Autodesk Inventor part; units mm, degrees
(part 4 of 4)
  spline S72 degree 5 poles (-3.5929, 3.9724) (-3.5942, 3.9738) (-3.5967, 3.9765) (-3.6006, 3.9805) (-3.6059, 3.9857) (-3.6128, 3.9919) (-3.6198, 3.998) (-3.627, 4.004) (-3.6342, 4.01) (-3.6414, 4.0159) (-3.6487, 4.0217) (-3.6561, 4.0275) (-3.6635, 4.0333) (-3.671, 4.039) (-3.6786, 4.0446) (-3.6863, 4.0501) (-3.694, 4.0556) (-3.7017, 4.061) (-3.7095, 4.0663) (-3.7174, 4.0716) (-3.7253, 4.0769) (-3.7333, 4.0821) (-3.7413, 4.0873) (-3.7493, 4.0925) (-3.7574, 4.0976) (-3.7656, 4.1026) (-3.7738, 4.1076) (-3.782, 4.1125) (-3.7903, 4.1174) (-3.7986, 4.1223) (-3.8069, 4.1271) (-3.8153, 4.1319) (-3.8237, 4.1367) (-3.8322, 4.1414) (-3.8407, 4.146) (-3.8493, 4.1507) (-3.8578, 4.1552) (-3.8665, 4.1598) (-3.8751, 4.1643) (-3.8838, 4.1688) (-3.8925, 4.1732) (-3.9013, 4.1776) (-3.9101, 4.182) (-3.9189, 4.1863) (-3.9278, 4.1906) (-3.9366, 4.1948) (-3.9456, 4.199) (-3.9545, 4.2032) (-3.9635, 4.2074) (-3.9725, 4.2115) (-3.9816, 4.2156) (-3.9907, 4.2196) (-3.9998, 4.2236) (-4.0089, 4.2276) (-4.0181, 4.2315) (-4.0273, 4.2354) (-4.0365, 4.2393) (-4.0458, 4.2431) (-4.0551, 4.2469) (-4.0644, 4.2507) (-4.0737, 4.2544) (-4.0831, 4.2581) (-4.0925, 4.2618) (-4.1019, 4.2654) (-4.1114, 4.269) (-4.1208, 4.2726) (-4.1304, 4.2761) (-4.1399, 4.2796) (-4.1533, 4.2845) (-4.1648, 4.2886) (-4.1744, 4.2919) (-4.1822, 4.2946) (-4.188, 4.2966) knots 0 0 0 0 0 0 0.014286 0.028571 0.042857 0.057143 0.071429 0.085714 0.1 0.114286 0.128571 0.142857 0.157143 0.171429 0.185714 0.2 0.214286 0.228571 0.242857 0.257143 0.271429 0.285714 0.3 0.314286 0.328571 0.342857 0.357143 0.371429 0.385714 0.4 0.414286 0.428571 0.442857 0.457143 0.471429 0.485714 0.5 0.514286 0.528571 0.542857 0.557143 0.571429 0.585714 0.6 0.614286 0.628571 0.642857 0.657143 0.671429 0.685714 0.7 0.714286 0.728571 0.742857 0.757143 0.771429 0.785714 0.8 0.814286 0.828571 0.842857 0.857143 0.871429 0.885714 0.9 0.914286 0.928571 0.942857 0.957143 1 1 1 1 1 1
  arc A73 (-4.188, 4.2966) -> (-4.3439, 4.1389) centre (0, 0) ccw
  spline S73 degree 5 poles (-4.013, 3.5476) (-4.0144, 3.5488) (-4.0171, 3.5513) (-4.0212, 3.5552) (-4.0264, 3.5604) (-4.0327, 3.5672) (-4.0389, 3.5742) (-4.045, 3.5813) (-4.051, 3.5884) (-4.057, 3.5956) (-4.0629, 3.6028) (-4.0688, 3.6101) (-4.0746, 3.6175) (-4.0804, 3.6249) (-4.0861, 3.6324) (-4.0917, 3.64) (-4.0972, 3.6477) (-4.1027, 3.6554) (-4.1082, 3.6631) (-4.1136, 3.6709) (-4.119, 3.6788) (-4.1243, 3.6867) (-4.1296, 3.6946) (-4.1348, 3.7026) (-4.14, 3.7106) (-4.1451, 3.7187) (-4.1502, 3.7269) (-4.1552, 3.735) (-4.1602, 3.7432) (-4.1652, 3.7515) (-4.1701, 3.7598) (-4.175, 3.7681) (-4.1798, 3.7765) (-4.1846, 3.7849) (-4.1894, 3.7934) (-4.1941, 3.8019) (-4.1988, 3.8104) (-4.2034, 3.819) (-4.208, 3.8276) (-4.2126, 3.8362) (-4.2172, 3.8449) (-4.2216, 3.8536) (-4.2261, 3.8623) (-4.2305, 3.8711) (-4.2349, 3.8799) (-4.2393, 3.8887) (-4.2436, 3.8976) (-4.2479, 3.9065) (-4.2521, 3.9155) (-4.2563, 3.9244) (-4.2605, 3.9334) (-4.2646, 3.9425) (-4.2688, 3.9515) (-4.2728, 3.9606) (-4.2769, 3.9698) (-4.2809, 3.9789) (-4.2848, 3.9881) (-4.2888, 3.9973) (-4.2927, 4.0066) (-4.2966, 4.0158) (-4.3004, 4.0251) (-4.3042, 4.0345) (-4.308, 4.0438) (-4.3117, 4.0532) (-4.3154, 4.0626) (-4.3191, 4.0721) (-4.3227, 4.0815) (-4.3264, 4.091) (-4.3314, 4.1043) (-4.3356, 4.1158) (-4.3391, 4.1254) (-4.3418, 4.1331) (-4.3439, 4.1389) knots 0 0 0 0 0 0 0.014286 0.028571 0.042857 0.057143 0.071429 0.085714 0.1 0.114286 0.128571 0.142857 0.157143 0.171429 0.185714 0.2 0.214286 0.228571 0.242857 0.257143 0.271429 0.285714 0.3 0.314286 0.328571 0.342857 0.357143 0.371429 0.385714 0.4 0.414286 0.428571 0.442857 0.457143 0.471429 0.485714 0.5 0.514286 0.528571 0.542857 0.557143 0.571429 0.585714 0.6 0.614286 0.628571 0.642857 0.657143 0.671429 0.685714 0.7 0.714286 0.728571 0.742857 0.757143 0.771429 0.785714 0.8 0.814286 0.828571 0.842857 0.857143 0.871429 0.885714 0.9 0.914286 0.928571 0.942857 0.957143 1 1 1 1 1 1
  line L73 (-3.9631, 3.5028) -> (-4.013, 3.5476)
  arc A74 (-3.9631, 3.5028) -> (-4.1449, 3.2856) centre (0, 0) ccw
  line L74 (-4.1449, 3.2856) -> (-4.1978, 3.3269)
  spline S74 degree 5 poles (-4.1978, 3.3269) (-4.1992, 3.328) (-4.2022, 3.3303) (-4.2067, 3.3336) (-4.2128, 3.3378) (-4.2206, 3.3429) (-4.2285, 3.3477) (-4.2365, 3.3524) (-4.2446, 3.3571) (-4.2528, 3.3617) (-4.2609, 3.3663) (-4.2691, 3.3708) (-4.2774, 3.3753) (-4.2858, 3.3797) (-4.2941, 3.3839) (-4.3026, 3.3881) (-4.3111, 3.3922) (-4.3197, 3.3963) (-4.3283, 3.4003) (-4.3369, 3.4042) (-4.3455, 3.4081) (-4.3543, 3.412) (-4.363, 3.4158) (-4.3718, 3.4195) (-4.3806, 3.4232) (-4.3895, 3.4268) (-4.3984, 3.4304) (-4.4073, 3.4339) (-4.4163, 3.4374) (-4.4253, 3.4409) (-4.4343, 3.4442) (-4.4434, 3.4476) (-4.4525, 3.4509) (-4.4616, 3.4541) (-4.4707, 3.4573) (-4.4799, 3.4605) (-4.4892, 3.4636) (-4.4984, 3.4667) (-4.5077, 3.4697) (-4.517, 3.4727) (-4.5263, 3.4756) (-4.5357, 3.4785) (-4.5451, 3.4814) (-4.5545, 3.4842) (-4.5639, 3.4869) (-4.5734, 3.4897) (-4.5829, 3.4924) (-4.5924, 3.495) (-4.602, 3.4976) (-4.6115, 3.5002) (-4.6211, 3.5027) (-4.6308, 3.5052) (-4.6404, 3.5077) (-4.6501, 3.5101) (-4.6598, 3.5124) (-4.6695, 3.5148) (-4.6792, 3.5171) (-4.689, 3.5193) (-4.6988, 3.5215) (-4.7086, 3.5237) (-4.7184, 3.5259) (-4.7283, 3.528) (-4.7381, 3.53) (-4.748, 3.5321) (-4.7579, 3.5341) (-4.7679, 3.536) (-4.7778, 3.5379) (-4.7878, 3.5398) (-4.8018, 3.5424) (-4.8139, 3.5446) (-4.8239, 3.5463) (-4.832, 3.5477) (-4.8381, 3.5487) knots 0 0 0 0 0 0 0.014286 0.028571 0.042857 0.057143 0.071429 0.085714 0.1 0.114286 0.128571 0.142857 0.157143 0.171429 0.185714 0.2 0.214286 0.228571 0.242857 0.257143 0.271429 0.285714 0.3 0.314286 0.328571 0.342857 0.357143 0.371429 0.385714 0.4 0.414286 0.428571 0.442857 0.457143 0.471429 0.485714 0.5 0.514286 0.528571 0.542857 0.557143 0.571429 0.585714 0.6 0.614286 0.628571 0.642857 0.657143 0.671429 0.685714 0.7 0.714286 0.728571 0.742857 0.757143 0.771429 0.785714 0.8 0.814286 0.828571 0.842857 0.857143 0.871429 0.885714 0.9 0.914286 0.928571 0.942857 0.957143 1 1 1 1 1 1
  arc A75 (-4.8381, 3.5487) -> (-4.9659, 3.3675) centre (0, 0) ccw
  spline S75 degree 5 poles (-4.5422, 2.8387) (-4.5437, 2.8397) (-4.5469, 2.8417) (-4.5515, 2.8448) (-4.5575, 2.8492) (-4.5649, 2.8548) (-4.5721, 2.8607) (-4.5793, 2.8666) (-4.5864, 2.8727) (-4.5935, 2.8788) (-4.6005, 2.8849) (-4.6075, 2.8912) (-4.6145, 2.8975) (-4.6214, 2.9039) (-4.6282, 2.9103) (-4.635, 2.9169) (-4.6418, 2.9235) (-4.6484, 2.9302) (-4.6551, 2.937) (-4.6617, 2.9438) (-4.6683, 2.9506) (-4.6748, 2.9575) (-4.6814, 2.9645) (-4.6878, 2.9715) (-4.6943, 2.9786) (-4.7006, 2.9857) (-4.707, 2.9929) (-4.7133, 3.0002) (-4.7196, 3.0074) (-4.7259, 3.0148) (-4.7321, 3.0221) (-4.7383, 3.0296) (-4.7444, 3.037) (-4.7505, 3.0445) (-4.7566, 3.0521) (-4.7627, 3.0597) (-4.7687, 3.0673) (-4.7747, 3.075) (-4.7807, 3.0827) (-4.7866, 3.0905) (-4.7925, 3.0983) (-4.7984, 3.1062) (-4.8042, 3.114) (-4.81, 3.122) (-4.8158, 3.1299) (-4.8215, 3.1379) (-4.8272, 3.146) (-4.8329, 3.1541) (-4.8386, 3.1622) (-4.8442, 3.1703) (-4.8498, 3.1785) (-4.8554, 3.1868) (-4.8609, 3.195) (-4.8665, 3.2033) (-4.8719, 3.2117) (-4.8774, 3.22) (-4.8828, 3.2284) (-4.8882, 3.2369) (-4.8936, 3.2454) (-4.8989, 3.2539) (-4.9043, 3.2624) (-4.9096, 3.271) (-4.9148, 3.2796) (-4.92, 3.2882) (-4.9253, 3.2969) (-4.9304, 3.3056) (-4.9356, 3.3144) (-4.9407, 3.3231) (-4.9478, 3.3355) (-4.9539, 3.3461) (-4.9589, 3.355) (-4.9629, 3.3621) (-4.9659, 3.3675) knots 0 0 0 0 0 0 0.014286 0.028571 0.042857 0.057143 0.071429 0.085714 0.1 0.114286 0.128571 0.142857 0.157143 0.171429 0.185714 0.2 0.214286 0.228571 0.242857 0.257143 0.271429 0.285714 0.3 0.314286 0.328571 0.342857 0.357143 0.371429 0.385714 0.4 0.414286 0.428571 0.442857 0.457143 0.471429 0.485714 0.5 0.514286 0.528571 0.542857 0.557143 0.571429 0.585714 0.6 0.614286 0.628571 0.642857 0.657143 0.671429 0.685714 0.7 0.714286 0.728571 0.742857 0.757143 0.771429 0.785714 0.8 0.814286 0.828571 0.842857 0.857143 0.871429 0.885714 0.9 0.914286 0.928571 0.942857 0.957143 1 1 1 1 1 1
  line L75 (-4.4856, 2.8027) -> (-4.5422, 2.8387)
  point P0 (0, 0)
  constraints: 152 end point, 152 point on circle, 76 centre point, 152 other
extrude "押し出し1" add sketch "スケッチ1" along normal blind 2.5
sketch "スケッチ2" plane through (2.5, 0, 0) normal (1, 0, 0) x (0, 0, -1)
  circle A0 centre (0, 0) radius 5.2892
  arc A1 (-2.0262, -4.8857) -> (-1.7617, -4.9872) centre (0, 0) ccw
  constraints: 1 centre point, 1 coincident, 1 concentric
extrude "押し出し2" add sketch "スケッチ2" along normal blind 3.5
sketch "スケッチ3" plane through (0, 0, 0) normal (-1, 0, 0) x (0, 0, 1)
  circle A0 centre (0, 0) radius 4.25
  dimension "d5" = 8.5
  constraints: 1 centre point, 1 coincident
  measures "d5" diameter of A0
extrude "押し出し3" cut sketch "スケッチ3" against normal blind 4
sketch "スケッチ4" plane through (4, 0, 0) normal (-1, 0, 0) x (0, 0, 1)
  circle A0 centre (0, 0) radius 1.5
  dimension "d8" = 3
  constraints: 1 centre point, 1 coincident
  measures "d8" diameter of A0
extrude "押し出し4" cut sketch "スケッチ4" against normal through all
sketch "スケッチ5" plane through (4, 0, 0) normal (-1, 0, 0) x (0, 0, 1)
  circle A0 centre (0, 0) radius 2
  circle A1 centre (0, 0) radius 1.5
  dimension "d11" = 4
  constraints: 1 centre point, 1 coincident
  measures "d11" diameter of A0
extrude "押し出し5" add sketch "スケッチ5" along normal blind 1.5
sketch "スケッチ6" plane through (6, 0, 0) normal (1, 0, 0) x (0, 0, -1)
  circle A0 centre (-3, 0) radius 0.875
  circle A1 centre (-1.5, -2.5981) radius 0.875
  circle A2 centre (1.5, -2.5981) radius 0.875
  circle A3 centre (3, 0) radius 0.875
  circle A4 centre (1.5, 2.5981) radius 0.875
  circle A5 centre (-1.5, 2.5981) radius 0.875
  point P0 (0, 0)
  point P1 (0, 0)
  point P2 (0, 0)
  point P3 (0, 0)
  point P4 (0, 0)
  point P5 (0, 0)
  dimension "d17" = 1.75
  dimension "d18" = 3
  dimension "d21" = 360
  constraints: 6 centre point, 2 coincident, 17 other
  measures "d17" diameter of A0
  measures "d18" distance of point (0, 0) A0.centre
extrude "押し出し6" cut sketch "スケッチ6" against normal through all
fillet "フィレット1" radius 1.5 1 edges at (4, 0, -2)
fillet "フィレット2" radius 0.3 1 edges at (2.5, 0, -2)
sketch "スケッチ7" plane through (6, 0, 0) normal (1, 0, 0) x (0, 0, -1)
  circle A0 centre (0, 0) radius 5.0392
  circle A1 centre (0, 0) radius 5.2892
  circle A2 centre (0, 0) radius 5.2892
  dimension "d27" = 0.25
  constraints: 2 centre point, 2 coincident, 1 concentric
  measures "d27" radial gap between concentric circles of A1 A0
extrude "押し出し7" cut sketch "スケッチ7" against normal up to surface (3.5 mm away)
